# Autodesk Inventor part: 大锥齿轮-主动轮
Saved by Autodesk Inventor 2015 (Build 190159000, 159)
## iProperties
Created: 2017-05-25
Part Number: 大锥齿轮-主动轮
Material: Steel, Mild
Document SubType Name: Modeling
Designer: Administrator
Categories: <?xml version="1.0" encoding="UTF-16"?> <MemberInstance><Categories><FamilyTemplate><FamilyTemplateParameter ValueType="xs:double" Id="1" ObjectReferenceKey="da_z" ObjectType="kUserParameterObject"/><FamilyTemplateParameter ValueType="xs:double" Id="2" ObjectReferenceKey="da_b" ObjectType="kUserParameterObject"/><FamilyTemplateParameter ValueType="xs:double" Id="3" ObjectReferenceKey="da_beta" ObjectType="kUserParameterObject"/><FamilyTemplateParameter ValueType="xs:double" Id="4" ObjectReferenceKey="da_dae" ObjectType="kUserParameterObject"/><FamilyTemplateParameter ValueType="xs:double" Id="5" ObjectReferenceKey="da_ve" ObjectType="kUserParameterObject"/><FamilyTemplateParameter ValueType="xs:double" Id="6" ObjectReferenceKey="da_omega" ObjectType="kUserParameterObject"/><FamilyTemplateParameter ValueType="xs:string" Id="7" ObjectReferenceKey="EAIAABAAAAAAHwAAAAAAAIAAAAAAAAAA" ObjectType="83914240" SubObjectId="SurfaceGeometry"/></FamilyTemplate><ParamToTemplateMap><ParamToTemplate CategoryParameter="//CategoryParameter[@InternalName='046C89C9-8512-4d59-83FE-43B91F4F132A']" TemplateParameter="1"/><ParamToTemplate CategoryParameter="//CategoryParameter[@InternalName='2552DF32-E462-4b46-AEBF-C6C7768E72AC']" TemplateParameter="2"/><ParamToTemplate CategoryParameter="//CategoryParameter[@InternalName='C9EE641D-15FC-4fae-A226-E94C4372FDD7']" TemplateParameter="3"/><ParamToTemplate><ParamToTemplate CategoryParameter="//CategoryParameter[@InternalName='00B6519A-459B-49c7-AD84-2E56D39A5744']" ConstantValue="0.000000"/></ParamToTemplate><ParamToTemplate><ParamToTemplate CategoryParameter="//CategoryParameter[@InternalName='04B31F0E-C7A6-4894-AA32-9629BEFACF47']" ConstantValue="1.000000"/></ParamToTemplate><ParamToTemplate><ParamToTemplate CategoryParameter="//CategoryParameter[@InternalName='43CBEC2E-7847-49e7-A936-2F7889FCB2D9']" ConstantValue="0.200000"/></ParamToTemplate><ParamToTemplate><ParamToTemplate CategoryParameter="//CategoryParameter[@InternalName='B1EFC894-105D-4ebd-86BF-FA20ED196853']" ConstantValue="0.300000"/></ParamToTemplate><ParamToTemplate><ParamToTemplate CategoryParameter="//CategoryParameter[@InternalName='51175063-3D10-4879-93E8-6246FE8B403D']" ConstantValue="2060000000.000000"/></ParamToTemplate><ParamToTemplate><ParamToTemplate CategoryParameter="//CategoryParameter[@InternalName='A3A52E27-4454-46a9-B0BD-C932399B70AF']" ConstantValue="0.300000"/></ParamToTemplate><ParamToTemplate CategoryParameter="//CategoryParameter[@InternalName='2A200944-5A8C-41ca-B96E-8520D2E510F1']" TemplateParameter="4"/><ParamToTemplate><ParamToTemplate CategoryParameter="//CategoryParameter[@InternalName='1A637F62-92C8-44bc-B81F-10802510B579']" ConstantValue="5.605440"/></ParamToTemplate><ParamToTemplate CategoryParameter="//CategoryParameter[@InternalName='B52DD4BE-6863-48fb-BF58-89EF6F9EC65C']" TemplateParameter="5"/><ParamToTemplate><ParamToTemplate CategoryParameter="//CategoryParameter[@InternalName='3956BFF2-84D2-457d-93C2-9B0613DEBA67']" ConstantValue="1.651925"/></ParamToTemplate><ParamToTemplate CategoryParameter="//CategoryParameter[@InternalName='739CFA02-461B-4bf8-8049-181FCAD8B28F']" TemplateParameter="6"/><ParamToTemplate><ParamToTemplate CategoryParameter="//CategoryParameter[@InternalName='A27E999F-E2CE-4481-8A2A-EBF499C4C3C5']" ConstantValue="0.000000"/></ParamToTemplate><ParamToTemplate><ParamToTemplate CategoryParameter="//CategoryParameter[@InternalName='9E1B4470-B2D3-4ff1-B813-535BB4CDF51A']" ConstantValue="3520000.000000"/></ParamToTemplate><ParamToTemplate><ParamToTemplate CategoryParameter="//CategoryParameter[@InternalName='F8452263-BFF6-458c-9FB1-07C4B99E95CD']" ConstantValue="11400000.000000"/></ParamToTemplate><ParamToTemplate><ParamToTemplate CategoryParameter="//CategoryParameter[@InternalName='3E3BB259-FD49-497f-8171-6EBC954A3479']" ConstantValue="2.000000"/></ParamToTemplate><ParamToTemplate CategoryParameter="//CategoryParameter[@InternalName='27C3BAF2-7550-4e4b-AE2C-0DB134B7D9B7']" TemplateParameter="7"/></ParamToTemplateMap><Category DisplayName="Gear" InternalName="DC85795E-93AB-48d5-8EEE-5A27447B64BD" Mnemonic="Gear"><CategoryParameter DisplayName="z" InternalName="046C89C9-8512-4d59-83FE-43B91F4F132A" Mnemonic="z"/><CategoryParameter DisplayName="b" InternalName="2552DF32-E462-4b46-AEBF-C6C7768E72AC" Mnemonic="b"/><CategoryParameter DisplayName="||b|" InternalName="C9EE641D-15FC-4fae-A226-E94C4372FDD7" Mnemonic="beta"/><CategoryParameter DisplayName="x" InternalName="00B6519A-459B-49c7-AD84-2E56D39A5744" Mnemonic="x"/><CategoryParameter DisplayName="a*" InternalName="04B31F0E-C7A6-4894-AA32-9629BEFACF47" Mnemonic="a"/><CategoryParameter DisplayName="c*" InternalName="43CBEC2E-7847-49e7-A936-2F7889FCB2D9" Mnemonic="c"/><CategoryParameter DisplayName="r|.f|*" InternalName="B1EFC894-105D-4ebd-86BF-FA20ED196853" Mnemonic="rf"/><CategoryParameter DisplayName="E" InternalName="51175063-3D10-4879-93E8-6246FE8B403D" Mnemonic="E"/><CategoryParameter DisplayName="||m|" InternalName="A3A52E27-4454-46a9-B0BD-C932399B70AF" Mnemonic="mi"/><Category DisplayName="BevelGear" InternalName="0C98F69A-0C2B-4791-B2FE-7691BB227E77" Mnemonic="BevelGear"><CategoryParameter DisplayName="d|.ae|" InternalName="2A200944-5A8C-41ca-B96E-8520D2E510F1" Mnemonic="dae"/><CategoryParameter DisplayName="d|.ai|" InternalName="1A637F62-92C8-44bc-B81F-10802510B579" Mnemonic="dai"/><CategoryParameter DisplayName="A|.e|" InternalName="B52DD4BE-6863-48fb-BF58-89EF6F9EC65C" Mnemonic="ve"/><CategoryParameter DisplayName="A|.i|" InternalName="3956BFF2-84D2-457d-93C2-9B0613DEBA67" Mnemonic="vi"/><CategoryParameter DisplayName="||S|" InternalName="739CFA02-461B-4bf8-8049-181FCAD8B28F" Mnemonic="omega"/><CategoryParameter DisplayName="x|.t|" InternalName="A27E999F-E2CE-4481-8A2A-EBF499C4C3C5" Mnemonic="xt"/><CategoryParameter DisplayName="||s||.Flim|" InternalName="9E1B4470-B2D3-4ff1-B813-535BB4CDF51A" Mnemonic="sFlim"/><CategoryParameter DisplayName="||s||.Hlim|" InternalName="F8452263-BFF6-458c-9FB1-07C4B99E95CD" Mnemonic="sHlim"/><CategoryParameter DisplayName="类型" InternalName="3E3BB259-FD49-497f-8171-6EBC954A3479" Mnemonic="type"/><CategoryParameter DisplayName="PitchDiameter" InternalName="27C3BAF2-7550-4e4b-AE2C-0DB134B7D9B7" Mnemonic="IDS_PITCHDIAM"/></Category></Category></Categories></MemberInstance>
Mass: 60.9118 g
Surface Area: 34.3074 cm^2
Volume: 7.7496 cm^3
Density: 7.86 g/cm^3
Appearance: Steel
CustomPartVersion: 1
Author: Administrator
Autodesk Inventor part; units mm, degrees
ref_plane "网格平面 2" through (0, 0, 0) normal (0.9945219, 0.1045285, 0) x (0, 0, 1)
sketch "齿实体草图" plane through (0, 0, 0) normal (1, 0, 0) x (0, 1, 0)
  line L0 (0, 0) -> (43.0031, -32.9954) construction
  line L1 (43.0031, -32.9954) -> (46.6641, -27.5038)
  line L2 (46.6641, -27.5038) -> (0, 0) construction
  line L3 (45, -30) -> (0, 0) construction
  line L4 (25.8283, -19.8175) -> (28.0272, -16.5192)
  line L5 (43.0031, -32.9954) -> (25.8283, -19.8175)
  line L6 (46.6641, -27.5038) -> (28.0272, -16.5192)
  line L7 (0, -39.3868) -> (0, 6.5645) projected
  line L8 (0, -30) -> (46.6641, -30) construction
  dimension "d0" = 90
  dimension "d1" = 86.0062
  dimension "d2" = 93.3282
  dimension "d3" = 21.6
  dimension "d4" = 27.5038
  constraints: 16 end point, 4 point on line, 3 perpendicular, 2 collinear, 1 horizontal alignment, 1 vertical alignment
  measures "d0" diameter of L3.start L7
  measures "d1" diameter of L0.end L7
  measures "d2" diameter of L1.end L7
  measures "d3" distance between parallel lines of L1 L4
  measures "d4" vertical distance of L1.end L0.start
revolve "齿实体" add sketch "齿实体草图" angle 360 about axis through (0, 0, 0) along (0, 0, 1)
ref_plane "齿平面" through (0, 45, -30) normal (0, -0.8320503, 0.5547002) x (1, 0, 0)
sketch "起始草图" plane through (0, 45, -30) normal (0, -0.8320503, 0.5547002) x (1, 0, 0)
  line L0 (0, -23.5051) -> (0, 10.6448) projected
  arc A0 (-1.064, -4.392) -> (-4.848, 4.8434) centre (-29.1857, -10.5213) ccw
  arc A1 (4.848, 4.8434) -> (1.064, -4.392) centre (29.1857, -10.5213) ccw
  line L1 (-1.064, -4.392) -> (1.064, -4.392)
  arc A2 (4.848, 4.8434) -> (-4.848, 4.8434) centre (0, -81.1249) ccw
  dimension "d7" = 28.7819
  dimension "d8" = 29.1857
  dimension "d9" = 70.6036
  dimension "d57" = 86.1049
  dimension "d58" = 76.7329
  constraints: 6 point on circle, 3 centre point, 3 symmetric about line, 2 end point, 1 coincident, 1 perpendicular, 1 other
  measures "d7" radius of A0
  measures "d8" horizontal distance of point (0, -81.125) A0.centre
  measures "d9" vertical distance of point (0, -81.125) A0.centre
  measures "d57" radius of A2
  measures "d58" distance from line of A2.centre L1
ref_plane "终止平面" through (0, 26.7531, -17.8354) normal (0, -0.8320503, 0.5547002) x (1, 0, 0)
sketch "终止草图" plane through (0, 26.7531, -17.8354) normal (0, -0.8320503, 0.5547002) x (1, 0, 0)
  line L0 (0, -15.3589) -> (0, 6.9827) projected
  arc A0 (-0.6336, -2.5344) -> (-2.887, 2.9654) centre (-17.3805, -6.1845) ccw
  arc A1 (2.887, 2.9654) -> (0.6336, -2.5344) centre (17.3805, -6.1845) ccw
  line L1 (-0.6336, -2.5344) -> (0.6336, -2.5344)
  arc A2 (2.887, 2.9654) -> (-2.887, 2.9654) centre (0, -48.2299) ccw
  dimension "d12" = 17.14
  dimension "d15" = 17.3805
  dimension "d16" = 42.0454
  dimension "d59" = 51.2767
  dimension "d60" = 45.6955
  constraints: 6 point on circle, 3 centre point, 3 symmetric about line, 2 end point, 1 coincident, 1 other
  measures "d12" radius of A0
  measures "d15" horizontal distance of A0.centre point (0, -48.23)
  measures "d16" vertical distance of A0.centre point (0, -48.23)
  measures "d59" radius of A2
  measures "d60" distance from line of A2.centre L1
loft "Loft" cut profiles "起始草图", "终止草图"
pattern_circular "Circular Pattern" count 30 over 360 about axis through (0, 0, 0) along (0, 0, 1) of "Loft"
sketch3d "三维草图 (右)"
ref_plane "终止平面 (右)" through (-5.881, 26.0987, -17.8354) normal (0.182904, -0.8116981, 0.5547002) x (0.9755397, 0.2198232, 0)
sketch "终止草图 (右)" plane through (-5.881, 26.0987, -17.8354) normal (0.182904, -0.8116981, 0.5547002) x (0.9755397, 0.2198232, 0)
  arc A0 (-0.6336, -2.5344) -> (-2.887, 2.9654) centre (-17.3805, -6.1845) ccw
  line L0 (0, -60.8319) -> (0, 16.393) projected
  arc A1 (2.887, 2.9654) -> (0.6336, -2.5344) centre (17.3805, -6.1845) ccw
  line L1 (-0.6336, -2.5344) -> (0.6336, -2.5344)
  arc A2 (2.887, 2.9654) -> (-2.887, 2.9654) centre (0, -48.2299) ccw
  dimension "d70" = 17.3805
  dimension "d71" = 42.0454
  dimension "d72" = 17.14
  dimension "d73" = 45.6955
  dimension "d74" = 51.2767
  constraints: 6 point on circle, 3 centre point, 3 symmetric about line, 2 end point, 1 coincident, 1 perpendicular, 1 other
  measures "d70" horizontal distance of A2.centre A0.centre
  measures "d71" vertical distance of point (0, -48.23) A0.centre
  measures "d72" radius of A0
  measures "d73" distance from line of point (0, -48.23) L1
  measures "d74" radius of A2
feature "放样 (右)" [suppressed]
pattern_circular "环形阵列 (右)" [suppressed]
sketch3d "三维草图 (左)"
ref_plane "终止平面 (左)" through (5.9165, 26.0987, -17.8526) normal (-0.1839159, -0.8112928, 0.5549586) x (0.9752545, -0.2210852, 0)
sketch "终止草图 (左)" plane through (5.9165, 26.0987, -17.8526) normal (-0.1839159, -0.8112928, 0.5549586) x (0.9752545, -0.2210852, 0)
  line L0 (0, -63.028) -> (0, 18.6015) projected
  arc A0 (-0.6336, -2.5244) -> (-2.887, 2.9754) centre (-17.3805, -6.1745) ccw
  arc A1 (2.887, 2.9754) -> (0.6336, -2.5244) centre (17.3805, -6.1745) ccw
  line L1 (-0.6336, -2.5244) -> (0.6336, -2.5244)
  ellipse E0 centre (0, -13.742) end of major axis (28.0272, -13.742) minor radius 15.5539 projected
  arc A2 (2.887, 2.9754) -> (-2.887, 2.9754) centre (0, -48.2199) ccw
  dimension "d56" = 15.5539
  dimension "d30" = 17.14
  dimension "d31" = 17.3805
  dimension "d32" = 42.0454
  dimension "d61" = 51.2767
  dimension "d62" = 45.6955
  constraints: 6 point on circle, 3 centre point, 3 symmetric about line, 2 end point, 1 coincident, 2 other
  measures "d30" radius of A0
  measures "d31" horizontal distance of point (0, -48.22) A0.centre
  measures "d32" vertical distance of A0.centre point (0, -48.22)
  measures "d61" radius of A2
  measures "d62" distance from line of point (0, -48.22) L1
feature "放样 (左)" [suppressed]
pattern_circular "环形阵列 (左)" [suppressed]
sketch "实体草图" plane through (0, 0, 0) normal (1, 0, 0) x (0, 1, 0)
  line L0 (0, -35.0375) -> (0, -19.5308) projected
  line L1 (43.0031, -32.9954) -> (25.8283, -19.8175) projected
  line L2 (25.8283, -19.8175) -> (0, -19.8175)
  line L3 (43.0031, -32.9954) -> (0, -32.9954)
  constraints: 4 end point, 2 perpendicular, 2 point on line
revolve "固定实体" add sketch "实体草图" angle 360 about axis through (0, 0, 0) along (0, 0, 1)
sketch "Sketch6" plane through (0, 0, 0) normal (1, 0, 0) x (0, 1, 0)
  line L0 (45, -30) -> (0, 0) projected
  line L1 (0, -37.7999) -> (0, 6.3) projected
surface revolve "中径" sketch "Sketch6" angle 360 about axis through (0, 0, 0) along (0, 0, 1) shown no curves L0
equation "\"d0\" = da_de"
equation "\"d1\" = da_dfe"
equation "\"d2\" = da_dae"
equation "\"d3\" = da_b"
equation "\"d4\" = da_ve"
equation "\"d7\" = fd_rr"
equation "\"d8\" = fd_x"
equation "\"d9\" = fd_y"
equation "\"d57\" = 0.5 * fd_dva + 0.3 * da_he"
equation "\"d58\" = 0.5 * fd_dva - 1.12 * da_he"
equation "\"da_teethtype\" = 0"
equation "\"da_b\" = 21.6"
equation "\"da_de\" = 90"
equation "\"da_dae\" = 93.3282"
equation "\"da_dfe\" = 86.00616"
equation "\"da_le\" = 54.08327"
equation "\"da_omega\" = 90deg"
equation "\"da_beta\" = 0"
equation "\"da_delta\" = 56.309932deg"
equation "\"da_alpha\" = 20deg"
equation "\"da_he\" = 6.6"
equation "\"da_ve\" = 27.50385"
equation "\"da_zv\" = 54.083269"
equation "\"fd_loft\" = da_b + 0.05 * da_he"
equation "\"fd_x\" = fd_x1 + fd_x2"
equation "\"fd_y\" = fd_y1 - fd_y2"
equation "\"fd_dd\" = fd_dva - 0.8 * da_he"
equation "\"da_dvw\" = 162.24981"
equation "\"d11\" = fd_loft"
equation "\"da_dm\" = 72.02771"
equation "\"da_x\" = 0"
equation "\"da_m\" = 3"
equation "\"d50\" = da_omega"
equation "\"fd_rr\" = 28.781931"
equation "\"fd_dva\" = 168.249807"
equation "\"fd_x1\" = 2.382032"
equation "\"fd_x2\" = 26.803654"
equation "\"fd_y1\" = 81.089925"
equation "\"fd_y2\" = 10.486355"
body "Solid1"
body "Srf1"
